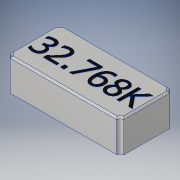
# Autodesk Inventor part: Crystal_ECX-34
Saved by Autodesk Inventor 2017 (Build 210142000, 142)
## iProperties
Created: 2016-08-15
Part Number: Crystal_ECX-34
Material: Aluminum 6061
Document SubType Name: Modeling
Designer: Bradley
Density: 2.7 g/cm^3
Appearance: Aluminum - Flat
Author: Bradley
Autodesk Inventor part; units mm, degrees
ref_plane "YZ Plane" through (0, 0, 0) normal (1, 0, 0) x (0, 1, 0)
ref_plane "XZ Plane" through (0, 0, 0) normal (0, 1, 0) x (-1, 0, 0)
ref_plane "XY Plane" through (0, 0, 0) normal (0, 0, 1) x (1, 0, 0)
sketch "Sketch1" plane through (0, 0, 0) normal (0, 1, 0) x (-1, 0, 0)
  line L0 (-1.6, 0.75) -> (1.6, 0.75)
  line L1 (1.6, 0.75) -> (1.6, -0.75)
  line L2 (1.6, -0.75) -> (-1.6, -0.75)
  line L3 (-1.6, -0.75) -> (-1.6, 0.75)
  line L4 (-1.6, 0.75) -> (1.6, -0.75) construction
  line L5 (1.6, 0.75) -> (-1.6, -0.75) construction
  arc A0 (1.6, -0.65) -> (1.5, -0.75) centre (1.6, -0.75) ccw
  arc A1 (-1.5, -0.75) -> (-1.6, -0.65) centre (-1.6, -0.75) ccw
  arc A2 (-1.6, 0.65) -> (-1.5, 0.75) centre (-1.6, 0.75) ccw
  arc A3 (1.5, 0.75) -> (1.6, 0.65) centre (1.6, 0.75) ccw
  point P0 (0, 0)
  dimension "d0" = 3.2
  dimension "d1" = 1.5
  dimension "d4" = 0.1
  constraints: 12 end point, 8 point on circle, 8 point on line, 4 centre point, 4 coincident, 3 equal radius, 2 midpoint, 2 parallel, 1 horizontal, 1 perpendicular
  measures "d0" distance of L1.end L2.end
  measures "d1" distance of L0.end L1.end
  measures "d4" radius of A0
extrude "Extrusion1" add sketch "Sketch1" along normal mid plane 0.9 contours L0 A3 L1 A0 L2 A1 L3 A2
chamfer "Chamfer1" distance 0.05 angle 45 8 edges at (0, 0.45, 0.75) (-1.5293, 0.45, 0.6793) (-1.6, 0.45, 0) (-1.5293, 0.45, -0.6793) (0, 0.45, -0.75) (1.5293, 0.45, -0.6793) (1.6, 0.45, 0) (1.5293, 0.45, 0.6793)
sketch "Sketch2" plane through (0, -0.45, 0) normal (0, -1, 0) x (1, 0, 0)
  line L0 (-1.6, 0.65) -> (-1.6, -0.65) projected
  arc A0 (-1.5, -0.75) -> (-1.6, -0.65) centre (-1.6, -0.75) ccw projected
  line L1 (-1.5, -0.75) -> (1.5, -0.75) projected
  arc A1 (1.6, -0.65) -> (1.5, -0.75) centre (1.6, -0.75) ccw projected
  line L2 (1.6, -0.65) -> (1.6, 0.65) projected
  arc A2 (1.5, 0.75) -> (1.6, 0.65) centre (1.6, 0.75) ccw projected
  line L3 (1.5, 0.75) -> (-1.5, 0.75) projected
  arc A3 (-1.6, 0.65) -> (-1.5, 0.75) centre (-1.6, 0.75) ccw projected
  arc A4 (-1.5, -0.75) -> (-1.6, -0.65) centre (-1.6, -0.75) ccw projected
  line L4 (-1.5741, -0.6534) -> (-1.5034, -0.5827)
  line L5 (-1.5034, -0.5827) -> (-1.5034, 0.5827)
  line L6 (-1.5034, 0.5827) -> (-1.5741, 0.6534)
  arc A5 (-1.6, 0.65) -> (-1.5, 0.75) centre (-1.6, 0.75) ccw projected
  line L7 (-1.5034, 0.7241) -> (-1.4327, 0.6534)
  line L8 (-1.4327, 0.6534) -> (-1.2, 0.6534)
  line L9 (-1.2, 0.6534) -> (-0.9, 0.3534)
  line L10 (-0.9, 0.3534) -> (-0.9, -0.6534)
  line L11 (-0.9, -0.6534) -> (-1.4327, -0.6534)
  line L12 (-1.4327, -0.6534) -> (-1.5034, -0.7241)
  arc A6 (1.5, 0.75) -> (1.6, 0.65) centre (1.6, 0.75) ccw projected
  line L13 (1.5034, 0.7241) -> (1.4327, 0.6534)
  line L14 (1.4327, 0.6534) -> (0.9, 0.6534)
  line L15 (0.9, 0.6534) -> (0.9, -0.6534)
  line L16 (0.9, -0.6534) -> (1.4327, -0.6534)
  line L17 (1.4327, -0.6534) -> (1.5034, -0.7241)
  arc A7 (1.6, -0.65) -> (1.5, -0.75) centre (1.6, -0.75) ccw projected
  line L18 (1.5741, -0.6534) -> (1.5034, -0.5827)
  line L19 (1.5034, -0.5827) -> (1.5034, 0.5827)
  line L20 (1.5034, 0.5827) -> (1.5741, 0.6534)
  line L21 (-1.6, 0.75) -> (-1.5293, 0.6793) construction
  line L22 (1.5, 0.75) -> (-1.5, 0.75) construction
  line L23 (-1.6, -0.75) -> (-1.5293, -0.6793) construction
  point P0 (0, 0)
  point P1 (0.9, 0)
  dimension "d8" = 1.8
  dimension "d9" = 0.1
  dimension "d10" = 0.3
  constraints: 38 end point, 15 point on circle, 9 equal length, 9 parallel, 7 perpendicular, 3 point on line, 1 collinear, 1 horizontal alignment, 1 midpoint, 1 vertical, 1 other
  measures "d8" distance between parallel lines of L15 L10
  measures "d9" distance between parallel lines of L6 L7
  measures "d10" horizontal distance of L8.end L9.end
extrude "Extrusion2" add sketch "Sketch2" along normal blind 0.01 contours A3 L7 L8 L9 L10 L11 L12 A0 L4 L5 L6 | A2 L20 L19 L18 A1 L17 L16 L15 L14 L13 | A2 L2 A1 L18 L19 L20
sketch "Sketch3" plane through (0, 0.45, 0) normal (0, 1, 0) x (1, 0, 0)
  line L0 (-1.4586, 0.7) -> (1.4586, 0.7) projected
  arc A0 (-1.55, 0.6086) -> (-1.4586, 0.7) centre (-1.6, 0.75) ccw projected
  line L1 (-1.55, -0.6086) -> (-1.55, 0.6086) projected
  arc A1 (-1.4586, -0.7) -> (-1.55, -0.6086) centre (-1.6, -0.75) ccw projected
  line L2 (1.4586, -0.7) -> (-1.4586, -0.7) projected
  arc A2 (1.55, -0.6086) -> (1.4586, -0.7) centre (1.6, -0.75) ccw projected
  line L3 (1.55, 0.6086) -> (1.55, -0.6086) projected
  arc A3 (1.4586, 0.7) -> (1.55, 0.6086) centre (1.6, 0.75) ccw projected
  line L4 (1.55, 0.6086) -> (1.55, -0.6086) construction
  line L5 (1.55, -0.3122) -> (-1.55, -0.3122) construction
  spline S0 degree 2 poles (-1.2875, 0.2309) (-1.3094, 0.2309) (-1.3527, 0.2202) (-1.3736, 0.212) knots 0 0 0 1 2 2 2
  spline S1 degree 2 poles (-1.3736, 0.212) (-1.393, 0.2037) (-1.4217, 0.1862) (-1.4329, 0.1784) knots 0 0 0 1 2 2 2
  line L6 (-1.4329, 0.1784) -> (-1.4378, 0.1784)
  line L7 (-1.4378, 0.1784) -> (-1.4378, 0.2635)
  spline S2 degree 2 poles (-1.4378, 0.2635) (-1.4115, 0.2776) (-1.3216, 0.3004) (-1.2812, 0.3004) knots 0 0 0 1 2 2 2
  spline S3 degree 2 poles (-1.2812, 0.3004) (-1.2404, 0.3004) (-1.1796, 0.2839) (-1.1548, 0.2664) knots 0 0 0 1 2 2 2
  spline S4 degree 2 poles (-1.1548, 0.2664) (-1.1285, 0.2474) (-1.1013, 0.1925) (-1.1013, 0.1556) knots 0 0 0 1 2 2 2
  spline S5 degree 2 poles (-1.1013, 0.1556) (-1.1013, 0.106) (-1.1665, 0.0311) (-1.2122, 0.0214) knots 0 0 0 1 2 2 2
  line L8 (-1.2122, 0.0214) -> (-1.2122, 0.0155)
  spline S6 degree 2 poles (-1.2122, 0.0155) (-1.1932, 0.0116) (-1.1499, -0.0059) (-1.1314, -0.0234) knots 0 0 0 1 2 2 2
  spline S7 degree 2 poles (-1.1314, -0.0234) (-1.113, -0.0404) (-1.0896, -0.0949) (-1.0896, -0.1342) knots 0 0 0 1 2 2 2
  spline S8 degree 2 poles (-1.0896, -0.1342) (-1.0896, -0.1746) (-1.1173, -0.2432) (-1.1426, -0.2694) knots 0 0 0 1 2 2 2
  spline S9 degree 2 poles (-1.1426, -0.2694) (-1.1689, -0.2966) (-1.2433, -0.3248) (-1.2904, -0.3248) knots 0 0 0 1 2 2 2
  spline S10 degree 2 poles (-1.2904, -0.3248) (-1.3357, -0.3248) (-1.4241, -0.303) (-1.4543, -0.2879) knots 0 0 0 1 2 2 2
  line L9 (-1.4543, -0.2879) -> (-1.4543, -0.2028)
  line L10 (-1.4543, -0.2028) -> (-1.4485, -0.2028)
  spline S11 degree 2 poles (-1.4485, -0.2028) (-1.4232, -0.2213) (-1.3376, -0.2553) (-1.2953, -0.2553) knots 0 0 0 1 2 2 2
  spline S12 degree 2 poles (-1.2953, -0.2553) (-1.2705, -0.2553) (-1.2209, -0.2397) (-1.2044, -0.2218) knots 0 0 0 1 2 2 2
  spline S13 degree 2 poles (-1.2044, -0.2218) (-1.1883, -0.2038) (-1.1713, -0.161) (-1.1713, -0.1284) knots 0 0 0 1 2 2 2
  spline S14 degree 2 poles (-1.1713, -0.1284) (-1.1713, -0.0958) (-1.1903, -0.0535) (-1.2073, -0.0414) knots 0 0 0 1 2 2 2
  spline S15 degree 2 poles (-1.2073, -0.0414) (-1.2243, -0.0292) (-1.2705, -0.02) (-1.2977, -0.02) knots 0 0 0 1 2 2 2
  line L11 (-1.2977, -0.02) -> (-1.3318, -0.02)
  line L12 (-1.3318, -0.02) -> (-1.3318, 0.0466)
  line L13 (-1.3318, 0.0466) -> (-1.305, 0.0466)
  spline S16 degree 2 poles (-1.305, 0.0466) (-1.2511, 0.0466) (-1.183, 0.0982) (-1.183, 0.1473) knots 0 0 0 1 2 2 2
  spline S17 degree 2 poles (-1.183, 0.1473) (-1.183, 0.1701) (-1.2005, 0.2027) (-1.2146, 0.2124) knots 0 0 0 1 2 2 2
  spline S18 degree 2 poles (-1.2146, 0.2124) (-1.2297, 0.2226) (-1.2666, 0.2309) (-1.2875, 0.2309) knots 0 0 0 1 2 2 2
  line L14 (-0.6292, -0.3122) -> (-0.9992, -0.3122)
  line L15 (-0.9992, -0.3122) -> (-0.9992, -0.2271)
  spline S19 degree 2 poles (-0.9992, -0.2271) (-0.9593, -0.1897) (-0.8883, -0.1201) (-0.8543, -0.0827) knots 0 0 0 1 2 2 2
  spline S20 degree 2 poles (-0.8543, -0.0827) (-0.7857, -0.0073) (-0.7357, 0.0831) (-0.7357, 0.1312) knots 0 0 0 1 2 2 2
  spline S21 degree 2 poles (-0.7357, 0.1312) (-0.7357, 0.1565) (-0.7512, 0.1944) (-0.7653, 0.2066) knots 0 0 0 1 2 2 2
  spline S22 degree 2 poles (-0.7653, 0.2066) (-0.7794, 0.2188) (-0.8164, 0.2309) (-0.8387, 0.2309) knots 0 0 0 1 2 2 2
  spline S23 degree 2 poles (-0.8387, 0.2309) (-0.8601, 0.2309) (-0.9039, 0.2202) (-0.9238, 0.212) knots 0 0 0 1 2 2 2
  spline S24 degree 2 poles (-0.9238, 0.212) (-0.9408, 0.2051) (-0.9724, 0.1857) (-0.9822, 0.1789) knots 0 0 0 1 2 2 2
  line L16 (-0.9822, 0.1789) -> (-0.9865, 0.1789)
  line L17 (-0.9865, 0.1789) -> (-0.9865, 0.2645)
  spline S25 degree 2 poles (-0.9865, 0.2645) (-0.9618, 0.2766) (-0.8728, 0.3004) (-0.8329, 0.3004) knots 0 0 0 1 2 2 2
  spline S26 degree 2 poles (-0.8329, 0.3004) (-0.7488, 0.3004) (-0.654, 0.2115) (-0.654, 0.1356) knots 0 0 0 1 2 2 2
  spline S27 degree 2 poles (-0.654, 0.1356) (-0.654, 0.1001) (-0.6705, 0.0408) (-0.6851, 0.0155) knots 0 0 0 1 2 2 2
  spline S28 degree 2 poles (-0.6851, 0.0155) (-0.6997, -0.0107) (-0.742, -0.0623) (-0.7653, -0.0871) knots 0 0 0 1 2 2 2
  spline S29 degree 2 poles (-0.7653, -0.0871) (-0.8032, -0.1284) (-0.8961, -0.2169) (-0.9238, -0.2427) knots 0 0 0 1 2 2 2
  line L18 (-0.9238, -0.2427) -> (-0.6292, -0.2427)
  line L19 (-0.6292, -0.2427) -> (-0.6292, -0.3122)
  line L20 (-0.4201, -0.3122) -> (-0.5164, -0.3122)
  line L21 (-0.5164, -0.3122) -> (-0.5164, -0.1974)
  line L22 (-0.5164, -0.1974) -> (-0.4201, -0.1974)
  line L23 (-0.4201, -0.1974) -> (-0.4201, -0.3122)
  line L24 (0.0778, 0.1979) -> (-0.1818, -0.3122)
  line L25 (-0.1818, -0.3122) -> (-0.2674, -0.3122)
  line L26 (-0.2674, -0.3122) -> (0.0068, 0.2173)
  line L27 (0.0068, 0.2173) -> (-0.3029, 0.2173)
  line L28 (-0.3029, 0.2173) -> (-0.3029, 0.2878)
  line L29 (-0.3029, 0.2878) -> (0.0778, 0.2878)
  line L30 (0.0778, 0.2878) -> (0.0778, 0.1979)
  spline S30 degree 2 poles (0.5305, -0.1177) (0.5305, -0.1639) (0.4998, -0.2422) (0.4741, -0.2684) knots 0 0 0 1 2 2 2
  spline S31 degree 2 poles (0.4741, -0.2684) (0.4473, -0.2962) (0.3802, -0.3248) (0.3399, -0.3248) knots 0 0 0 1 2 2 2
  spline S32 degree 2 poles (0.3399, -0.3248) (0.2995, -0.3248) (0.2329, -0.2976) (0.2076, -0.2704) knots 0 0 0 1 2 2 2
  spline S33 degree 2 poles (0.2076, -0.2704) (0.1765, -0.2378) (0.1415, -0.1284) (0.1415, -0.0487) knots 0 0 0 1 2 2 2
  spline S34 degree 2 poles (0.1415, -0.0487) (0.1415, 0.0296) (0.1736, 0.1556) (0.2071, 0.2022) knots 0 0 0 1 2 2 2
  spline S35 degree 2 poles (0.2071, 0.2022) (0.2397, 0.2479) (0.3428, 0.299) (0.4104, 0.299) knots 0 0 0 1 2 2 2
  spline S36 degree 2 poles (0.4104, 0.299) (0.4303, 0.299) (0.4653, 0.2951) (0.4784, 0.2907) knots 0 0 0 1 2 2 2
  line L31 (0.4784, 0.2907) -> (0.4784, 0.2134)
  line L32 (0.4784, 0.2134) -> (0.475, 0.2134)
  spline S37 degree 2 poles (0.475, 0.2134) (0.4639, 0.2192) (0.423, 0.2295) (0.3997, 0.2295) knots 0 0 0 1 2 2 2
  spline S38 degree 2 poles (0.3997, 0.2295) (0.3248, 0.2295) (0.2329, 0.1283) (0.2241, 0.0291) knots 0 0 0 1 2 2 2
  spline S39 degree 2 poles (0.2241, 0.0291) (0.2528, 0.0491) (0.3131, 0.0709) (0.3491, 0.0709) knots 0 0 0 1 2 2 2
  spline S40 degree 2 poles (0.3491, 0.0709) (0.3841, 0.0709) (0.4366, 0.0568) (0.4653, 0.0355) knots 0 0 0 1 2 2 2
  spline S41 degree 2 poles (0.4653, 0.0355) (0.4984, 0.0107) (0.5305, -0.0662) (0.5305, -0.1177) knots 0 0 0 1 2 2 2
  spline S42 degree 2 poles (0.4488, -0.1211) (0.4488, -0.0842) (0.4293, -0.0341) (0.4079, -0.0166) knots 0 0 0 1 2 2 2
  spline S43 degree 2 poles (0.4079, -0.0166) (0.3919, -0.0039) (0.352, 0.0043) (0.3311, 0.0043) knots 0 0 0 1 2 2 2
  spline S44 degree 2 poles (0.3311, 0.0043) (0.3029, 0.0043) (0.2499, -0.0127) (0.2241, -0.0287) knots 0 0 0 1 2 2 2
  spline S45 degree 2 poles (0.2241, -0.0287) (0.2237, -0.0375) (0.2227, -0.054) (0.2227, -0.0667) knots 0 0 0 1 2 2 2
  spline S46 degree 2 poles (0.2227, -0.0667) (0.2227, -0.1289) (0.247, -0.2052) (0.2655, -0.2252) knots 0 0 0 1 2 2 2
  spline S47 degree 2 poles (0.2655, -0.2252) (0.2825, -0.2441) (0.3194, -0.2592) (0.3404, -0.2592) knots 0 0 0 1 2 2 2
  spline S48 degree 2 poles (0.3404, -0.2592) (0.389, -0.2592) (0.4488, -0.1902) (0.4488, -0.1211) knots 0 0 0 1 2 2 2
  spline S49 degree 2 poles (0.7828, -0.3258) (0.7381, -0.3258) (0.6647, -0.2991) (0.6389, -0.2743) knots 0 0 0 1 2 2 2
  spline S50 degree 2 poles (0.6389, -0.2743) (0.6136, -0.25) (0.5874, -0.1838) (0.5874, -0.1464) knots 0 0 0 1 2 2 2
  spline S51 degree 2 poles (0.5874, -0.1464) (0.5874, -0.0978) (0.6394, -0.0161) (0.689, 0.0082) knots 0 0 0 1 2 2 2
  line L33 (0.689, 0.0082) -> (0.689, 0.0107)
  spline S52 degree 2 poles (0.689, 0.0107) (0.6447, 0.0364) (0.6019, 0.0977) (0.6019, 0.1434) knots 0 0 0 1 2 2 2
  spline S53 degree 2 poles (0.6019, 0.1434) (0.6019, 0.211) (0.7041, 0.3014) (0.7828, 0.3014) knots 0 0 0 1 2 2 2
  spline S54 degree 2 poles (0.7828, 0.3014) (0.8645, 0.3014) (0.9632, 0.2158) (0.9632, 0.1487) knots 0 0 0 1 2 2 2
  spline S55 degree 2 poles (0.9632, 0.1487) (0.9632, 0.1084) (0.916, 0.0296) (0.8718, 0.0073) knots 0 0 0 1 2 2 2
  line L34 (0.8718, 0.0073) -> (0.8718, 0.0048)
  spline S56 degree 2 poles (0.8718, 0.0048) (0.9243, -0.0195) (0.9783, -0.0895) (0.9783, -0.1449) knots 0 0 0 1 2 2 2
  spline S57 degree 2 poles (0.9783, -0.1449) (0.9783, -0.2218) (0.8665, -0.3258) (0.7828, -0.3258) knots 0 0 0 1 2 2 2
  spline S58 degree 2 poles (0.8956, -0.1527) (0.8956, -0.1158) (0.8665, -0.072) (0.8251, -0.0496) knots 0 0 0 1 2 2 2
  spline S59 degree 2 poles (0.8251, -0.0496) (0.8115, -0.0419) (0.7658, -0.0239) (0.7371, -0.0122) knots 0 0 0 1 2 2 2
  spline S60 degree 2 poles (0.7371, -0.0122) (0.7041, -0.0341) (0.6686, -0.0992) (0.6686, -0.1406) knots 0 0 0 1 2 2 2
  spline S61 degree 2 poles (0.6686, -0.1406) (0.6686, -0.195) (0.7342, -0.266) (0.7838, -0.266) knots 0 0 0 1 2 2 2
  spline S62 degree 2 poles (0.7838, -0.266) (0.8344, -0.266) (0.8956, -0.2052) (0.8956, -0.1527) knots 0 0 0 1 2 2 2
  spline S63 degree 2 poles (0.8844, 0.1478) (0.8844, 0.1881) (0.8305, 0.2421) (0.7823, 0.2421) knots 0 0 0 1 2 2 2
  spline S64 degree 2 poles (0.7823, 0.2421) (0.7386, 0.2421) (0.6827, 0.194) (0.6827, 0.1526) knots 0 0 0 1 2 2 2
  spline S65 degree 2 poles (0.6827, 0.1526) (0.6827, 0.123) (0.7113, 0.0816) (0.74, 0.0651) knots 0 0 0 1 2 2 2
  spline S66 degree 2 poles (0.74, 0.0651) (0.7522, 0.0583) (0.8037, 0.0345) (0.8246, 0.0277) knots 0 0 0 1 2 2 2
  spline S67 degree 2 poles (0.8246, 0.0277) (0.8596, 0.0544) (0.8844, 0.1113) (0.8844, 0.1478) knots 0 0 0 1 2 2 2
  line L35 (1.5063, -0.3122) -> (1.4028, -0.3122)
  line L36 (1.4028, -0.3122) -> (1.1835, -0.0331)
  line L37 (1.1835, -0.0331) -> (1.1485, -0.0725)
  line L38 (1.1485, -0.0725) -> (1.1485, -0.3122)
  line L39 (1.1485, -0.3122) -> (1.0687, -0.3122)
  line L40 (1.0687, -0.3122) -> (1.0687, 0.2878)
  line L41 (1.0687, 0.2878) -> (1.1485, 0.2878)
  line L42 (1.1485, 0.2878) -> (1.1485, 0.0121)
  line L43 (1.1485, 0.0121) -> (1.3945, 0.2878)
  line L44 (1.3945, 0.2878) -> (1.4917, 0.2878)
  line L45 (1.4917, 0.2878) -> (1.2433, 0.0199)
  line L46 (1.2433, 0.0199) -> (1.5063, -0.3122)
  point P0 (0, 0)
  constraints: 2 end point, 2 point on line, 1 horizontal, 1 perpendicular
extrude "Extrusion3" add sketch "Sketch3" along normal blind 0.01 contours S0 S1 L6 L7 S2 S3 S4 S5 L8 S6 S7 S8 S9 S10 L9 L10 S11 S12 S13 S14 S15 L11 L12 L13 S16 S17 S18 | L14 L15 S19 S20 S21 S22 S23 S24 L16 L17 S25 S26 S27 S28 S29 L18 L19 | L20 L21 L22 L23 | L24 L25 L26 L27 L28 L29 L30 | S30 S31 S32 S33 S34 S35 S36 L31 L32 S37 S38 S39 S40 S41 | S49 S50 S51 L33 S52 S53 S54 S55 L34 S56 S57 | L35 L36 L37 L38 L39 L40 L41 L42 L43 L44 L45 L46
body "Solid1"
